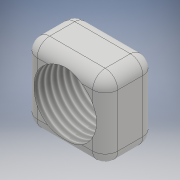
# Autodesk Inventor part: benzcadnut
Saved by Autodesk Inventor 2017 (Build 210142000, 142)
## iProperties
Created: 2018-03-01
Part Number: benzcadnut
Material: Generic
Document SubType Name: Modeling
Designer: CMRU-CAD-PC 02
Density: 1 g/cm^3
Appearance: Default
Author: CMRU-CAD-PC 02
Autodesk Inventor part; units mm, degrees
ref_plane "YZ Plane" through (0, 0, 0) normal (1, 0, 0) x (0, 1, 0)
ref_plane "XZ Plane" through (0, 0, 0) normal (0, 1, 0) x (-1, 0, 0)
ref_plane "XY Plane" through (0, 0, 0) normal (0, 0, 1) x (1, 0, 0)
sketch "Sketch1" plane through (0, 0, 0) normal (0, 1, 0) x (-1, 0, 0)
  circle A0 centre (0, 0) radius 5
  line L0 (6.4276, 6.2219) -> (-6.4276, 6.2219)
  line L1 (-6.4276, 6.2219) -> (-6.4276, -6.2219)
  line L2 (-6.4276, -6.2219) -> (6.4276, -6.2219)
  line L3 (6.4276, -6.2219) -> (6.4276, 6.2219)
  line L4 (6.4276, 6.2219) -> (-6.4276, -6.2219) construction
  line L5 (-6.4276, 6.2219) -> (6.4276, -6.2219) construction
  dimension "d0" = 10
  constraints: 12 end point, 2 midpoint, 2 parallel, 1 centre point, 1 coincident, 1 horizontal, 1 perpendicular
  measures "d0" diameter of A0
extrude "Extrusion1" add sketch "Sketch1" along normal blind 8
fillet "Fillet1" radius 2 12 edges at (6.4276, 8, 0) (0, 8, -6.2219) (0, 8, 6.2219) (-6.4276, 8, 0) (-6.4276, 0, 0) (0, 0, 6.2219) (6.4276, 0, 0) (0, 0, -6.2219) (-6.4276, 4, -6.2219) (6.4276, 4, 6.2219) (6.4276, 4, -6.2219) (-6.4276, 4, 6.2219)
thread "Thread1" size "M10x1" class "6H" standard "ANSI Metric M Profile" full length
body "Solid1"
